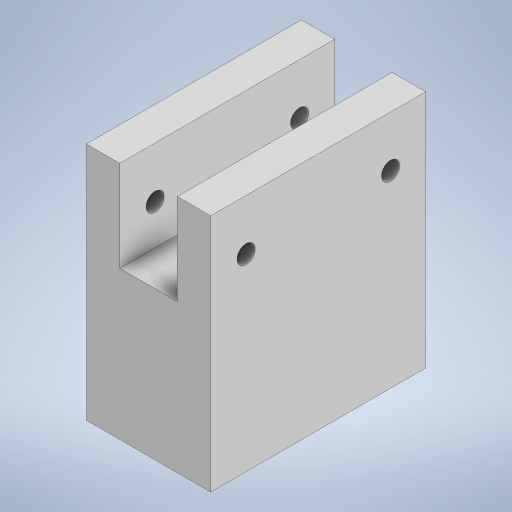
# Autodesk Inventor part: housing
Saved by Autodesk Inventor 2024.3 (Build 283343000, 343)
## iProperties
Created: 2025-07-08
Part Number: housing
Material: Generic
Document SubType Name: Modeling
Designer: user
Density: 1 g/cm^3
Appearance: Default
Author: user
Autodesk Inventor part; units mm, degrees
ref_plane "YZ Plane" through (0, 0, 0) normal (1, 0, 0) x (0, 1, 0)
ref_plane "XZ Plane" through (0, 0, 0) normal (0, 1, 0) x (-1, 0, 0)
ref_plane "XY Plane" through (0, 0, 0) normal (0, 0, 1) x (1, 0, 0)
sketch "Sketch1" plane through (0, 0, 0) normal (0, 1, 0) x (-1, 0, 0)
  line L0 (-13, 22.45) -> (13, 22.45)
  line L1 (13, 22.45) -> (13, -22.45)
  line L2 (13, -22.45) -> (-13, -22.45)
  line L3 (-13, -22.45) -> (-13, 22.45)
  line L4 (-13, 22.45) -> (13, -22.45) construction
  line L5 (13, 22.45) -> (-13, -22.45) construction
  point P0 (0, 0)
  dimension "d0" = 26
  dimension "d1" = 44.9
  constraints: 12 end point, 2 midpoint, 2 parallel, 1 horizontal, 1 perpendicular
  measures "d0" distance of L1.end L2.end
  measures "d1" distance of L0.end L1.end
extrude "Extrusion1" add sketch "Sketch1" along normal blind 50
sketch "Sketch2" plane through (-13, 0, 22.45) normal (0, 0, 1) x (1, 0, 0)
  line L0 (0, 0) -> (26, 0) projected
  line L1 (26, 0) -> (26, 50) projected
  line L2 (0, 50) -> (26, 50) projected
  line L3 (0, 0) -> (0, 50) projected
  line L4 (13, 50) -> (13, 0)
  line L5 (13, 50) -> (7, 50)
  line L6 (26, 50) -> (0, 50) projected
  line L7 (7, 50) -> (7, 31)
  line L8 (7, 31) -> (19, 31)
  line L9 (19, 31) -> (19, 50)
  line L10 (13, 50) -> (19, 50)
  dimension "d4" = 6
  dimension "d5" = 19
  dimension "d6" = 12
  constraints: 12 end point, 2 perpendicular, 2 point on line, 2 vertical, 1 collinear, 1 midpoint
  measures "d4" distance of L4.start L5.end
  measures "d5" distance of L5.end L7.end
  measures "d6" distance of L7.end L8.end
extrude "Extrusion2" cut sketch "Sketch2" against normal blind 50 contours L8 L7 L2 L4 | L4 L2 L9 L8
sketch "Sketch3" plane through (13, 0, 22.45) normal (1, 0, 0) x (0, 0, -1)
  circle A0 centre (7.35, 39.4) radius 1.9
  circle A1 centre (37.55, 39.4) radius 1.9
  line L0 (0, 50) -> (44.9, 50) projected
  line L1 (22.45, 50) -> (22.45, 0)
  line L2 (44.9, 0) -> (0, 0) projected
  point P0 (22.45, 25)
  point P1 (3.8014, 50)
  dimension "d9" = 3.8
  constraints: 2 centre point, 2 end point, 2 midpoint, 1 perpendicular, 1 point on line
  measures "d9" diameter of A0
extrude "Extrusion3" cut sketch "Sketch3" against normal blind 50
body "Solid1"
